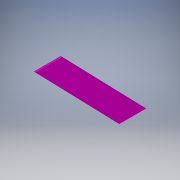
# Autodesk Inventor part: Cross Brace
Saved by Autodesk Inventor 2017 (Build 210142000, 142)
## iProperties
Created: 2017-01-26
Part Number: Cross Brace
Material: Generic
Document SubType Name: Modeling
Designer: Ben
Density: 1 g/cm^3
Appearance: Magenta
Author: Ben
Autodesk Inventor part; units mm, degrees
ref_plane "YZ Plane" through (0, 0, 0) normal (1, 0, 0) x (0, 1, 0)
ref_plane "XZ Plane" through (0, 0, 0) normal (0, 1, 0) x (-1, 0, 0)
ref_plane "XY Plane" through (0, 0, 0) normal (0, 0, 1) x (1, 0, 0)
sketch "Sketch1" plane through (0, 0, 0) normal (1, 0, 0) x (0, 1, 0)
  line L0 (165.1, 185.3184) -> (165.1, 134.5184)
  line L1 (165.1, 134.5184) -> (0, -25.4)
  line L2 (0, -25.4) -> (0, 25.4)
  line L3 (0, 25.4) -> (165.1, 185.3184)
  line L4 (0, 0) -> (26.223, 0) construction
  line L5 (165.1, 159.9184) -> (138.877, 159.9184) construction
  line L6 (0, 25.4) -> (52.446, 25.4) construction
  line L7 (165.1, 134.5184) -> (112.654, 134.5184) construction
  circle A0 centre (158.75, 166.2684) radius 1.5875
  line L8 (165.1, 147.2184) -> (125.7655, 147.2184) construction
  line L9 (165.1, 166.2684) -> (145.4328, 166.2684) construction
  line L10 (158.75, 166.2684) -> (158.75, 147.2184) construction
  circle A1 centre (158.75, 147.2184) radius 1.5875
  circle A2 centre (139.7, 147.2184) radius 1.5875
  line L11 (0, -6.35) -> (19.6672, -6.35) construction
  line L12 (39.3345, 12.7) -> (0, 12.7) construction
  line L13 (6.35, -6.35) -> (6.35, 12.7) construction
  circle A3 centre (6.35, -6.35) radius 1.5875
  circle A4 centre (6.35, 12.7) radius 1.5875
  circle A5 centre (25.4, 12.7) radius 1.5875
  point P0 (0, 0)
  dimension "d0" = 50.8
  dimension "d4" = 159.9184
  dimension "d5" = 3.175
  dimension "d6" = 19.05
  dimension "d7" = 6.35
  dimension "d8" = 19.05
  dimension "d9" = 6.35
  dimension "d10" = 19.05
  dimension "d11" = 6.35
  dimension "d12" = 6.35
  dimension "d13" = 19.05
  dimension "d16" = 152.4
  constraints: 28 end point, 18 point on line, 6 centre point, 6 horizontal, 5 equal radius, 4 coincident, 3 parallel, 3 perpendicular, 2 midpoint, 1 vertical
  measures "d0" distance of L1.end L2.end
  measures "d4" distance between parallel lines of L4 L5
  measures "d5" diameter of A0
  measures "d6" distance of L10.start L10.end
  measures "d7" distance between parallel lines of L0 L10
  measures "d8" distance of A2.centre L10.end
  measures "d9" distance from line of L5 L10.start
  measures "d10" distance of L13.start L13.end
  measures "d11" distance between parallel lines of L4 L11
  measures "d12" distance between parallel lines of L13 L2
  measures "d13" distance of L13.end A5.centre
  measures "d16" distance between parallel lines of L10 L13
extrude "Extrusion1" add sketch "Sketch1" along normal blind 3.175
body "Solid1"
